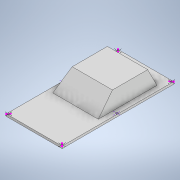
# Autodesk Inventor part: Karosserie_Abdeckung
Saved by Autodesk Inventor 2021 (Build 250183000, 183)
## iProperties
Created: 2021-01-27
Part Number: Karosserie_Abdeckung
Material: Generisch
Document SubType Name: Modeling
Designer: Jaro Machnow
Density: 1 g/cm^3
Appearance: Vorgabe
Author: Jaro Machnow
Autodesk Inventor part; units mm, degrees
ref_plane "YZ Plane" through (0, 0, 0) normal (1, 0, 0) x (0, 1, 0)
ref_plane "XZ Plane" through (0, 0, 0) normal (0, 1, 0) x (-1, 0, 0)
sketch "Skizze1" plane through (0, 0, 0) normal (0, 1, 0) x (-1, 0, 0)
  line L0 (125, 250) -> (-125, 250)
  line L1 (-125, 250) -> (-125, -250)
  line L2 (-125, -250) -> (125, -250)
  line L3 (125, -250) -> (125, 250)
  line L4 (0, 250) -> (0, -250) construction
  line L5 (125, 0) -> (-125, 0) construction
  point P0 (0, 0)
  point P1 (0, 0)
  dimension "d0" = 250
  dimension "d1" = 500
  constraints: 12 end point, 6 midpoint, 2 parallel, 1 horizontal, 1 perpendicular
  measures "d0" distance of L2.end L1.end
  measures "d1" distance of L1.end L0.end
extrude "Extrusion1" add sketch "Skizze1" along normal blind 10
sketch "Skizze2" plane through (0, 10, 0) normal (0, 1, 0) x (1, 0, 0)
  line L0 (-101.9878, -64.7205) -> (101.9878, -64.7205)
  line L1 (101.9878, -64.7205) -> (101.9878, 197.9709)
  line L2 (101.9878, 197.9709) -> (-101.9878, 197.9709)
  line L3 (-101.9878, 197.9709) -> (-101.9878, -64.7205)
  line L4 (0, -64.7205) -> (0, 197.9709) construction
  line L5 (-125, -250) -> (125, -250) construction
  line L6 (0, -250) -> (0, 250) construction
  line L7 (125, 250) -> (-125, 250) construction
  line L8 (-125, 250) -> (-125, -250) projected
  point P0 (0, 0)
  point P1 (0, 0)
  point P2 (-125, 0)
  constraints: 12 end point, 6 midpoint, 2 parallel, 1 horizontal, 1 perpendicular, 1 point on line
ref_plane "Arbeitsebene1" through (0, 80, 0) normal (0, 1, 0) x (1, 0, 0)
sketch "Skizze3" plane through (0, 80, 0) normal (0, 1, 0) x (1, 0, 0)
  line L0 (-90.1948, 10.416) -> (90.1948, 10.416)
  line L1 (90.1948, 10.416) -> (90.1948, 168.2192)
  line L2 (90.1948, 168.2192) -> (-90.1948, 168.2192)
  line L3 (-90.1948, 168.2192) -> (-90.1948, 10.416)
  line L4 (0, 10.416) -> (0, 168.2192) construction
  line L5 (-125, -250) -> (125, -250) construction
  line L6 (0, -250) -> (0, 250) construction
  line L7 (125, 250) -> (-125, 250) construction
  point P0 (0, 0)
  point P1 (0, 0)
  point P2 (0, 0)
  constraints: 16 end point, 5 midpoint, 2 parallel, 1 horizontal, 1 perpendicular, 1 point on line
loft "Erhebung1" add profiles "Skizze2", "Skizze3"
shell "Wandung1" thickness 10 removed faces 1 at (41.6667, 0, 83.3333)
sketch "Skizze4" plane through (0, 10, 0) normal (0, 1, 0) x (1, 0, 0)
  line L0 (-125, -250) -> (-115, -240) projected
  line L1 (-125, 250) -> (-115, 240) projected
  line L2 (125, 250) -> (115, 240) projected
  line L3 (125, -250) -> (115, -240) projected
  point P0 (0, 0)
  point P1 (-120, -245)
  point P2 (-120, 245)
  point P3 (120, 245)
  point P4 (120, -245)
  point P5 (-120, 0)
  point P6 (120, 0)
  constraints: 4 midpoint
sketch "Skizze5" plane through (0, 10, 0) normal (0, 1, 0) x (1, 0, 0)
  point P0 (120, -245)
  point P1 (-120, -245)
  point P2 (-120, 245)
  point P3 (120, 245)
  point P4 (-120, 0)
  point P5 (120, 0)
hole "Bohrung1" at (120, 10, 245) at (-120, 10, 245) at (-120, 10, -245) at (120, 10, -245) at (-120, 10, 0) at (120, 10, 0) direction (0, -1, 0) diameter 5.5 end through all countersink diameter 10.4 countersink angle 90
equation "\"d0\" = 0.5 * d1"
